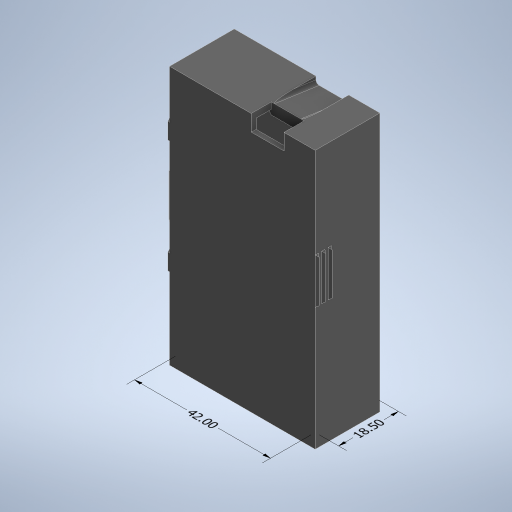
# Autodesk Inventor part: battery
Saved by Autodesk Inventor 2024.1 (Build 281209000, 209)
## iProperties
Created: 2025-03-04
Part Number: battery
Material: 一般
Document SubType Name: Modeling
Designer: hibik
Density: 1 g/cm^3
Appearance: 既定
Author: hibik
Autodesk Inventor part; units mm, degrees
sketch "スケッチ1" plane through (0, 0, 0) normal (0, 1, 0) x (-1, 0, 0)
  line L0 (-22.5, -10) -> (22.5, -10)
  line L1 (22.5, -10) -> (22.5, 10)
  line L2 (22.5, 10) -> (-22.5, 10)
  line L3 (-22.5, 10) -> (-22.5, -10)
  line L4 (-22.5, -10) -> (22.5, 10) construction
  line L5 (22.5, -10) -> (-22.5, 10) construction
  point P0 (0, 0)
  dimension "d0" = 45
  dimension "d1" = 20
  constraints: 12 end point, 2 midpoint, 2 parallel, 1 horizontal, 1 perpendicular
  measures "d0" distance of L2.end L1.end
  measures "d1" distance of L1.end L0.end
extrude "押し出し1" add sketch "スケッチ1" along normal blind 90
sketch "スケッチ2" plane through (-22.5, 0, 10) normal (0, 0, 1) x (1, 0, 0)
  line L0 (0, 0) -> (0, 90) projected
  line L1 (0, 65) -> (-3, 65)
  line L2 (-3, 65) -> (-3, 60)
  line L3 (-3, 60) -> (0, 60)
  line L4 (0, 60) -> (0, 65)
  line L5 (-3, 67.5) -> (-5, 67.5)
  line L6 (-5, 67.5) -> (-5, 57.5)
  line L7 (-5, 57.5) -> (-3, 57.5)
  line L8 (-3, 57.5) -> (-3, 67.5)
  line L9 (0, 90) -> (45, 90) projected
  point P0 (22.5, 0)
  point P1 (-5, 62.5)
  point P2 (-3, 62.5)
  point P3 (-3, 60)
  point P4 (0, 60)
  point P5 (-3, 65)
  dimension "d14" = 5
  dimension "d15" = 10
  dimension "d16" = 2
  dimension "d17" = 3
  dimension "d18" = 25
  constraints: 16 end point, 4 parallel, 2 horizontal, 2 midpoint, 2 perpendicular, 1 collinear, 1 horizontal alignment, 1 point on line
  measures "d14" distance of L1.end L2.end
  measures "d15" distance of L5.end L6.end
  measures "d16" distance of L5.start L5.end
  measures "d17" distance of L1.start L1.end
  measures "d18" distance between parallel lines of L9 L1
ref_plane "作業平面1" through (0, 45, 0) normal (0, 1, 0) x (1, 0, 0)
extrude "押し出し2" add sketch "スケッチ2" against normal up to surface (20 mm away)
mirror "ミラー1" about plane through (0, 45, 0) normal (0, 1, 0) of "押し出し2"
sketch "スケッチ3" plane through (-27.5, 67.5, 10) normal (0, 1, 0) x (1, 0, 0)
  line L0 (4.5, 0) -> (-25.5, 51.9615) projected
  line L1 (2, 20) -> (0, 20) projected
  line L2 (0, 0) -> (0, 20) projected
  line L3 (2, 0) -> (0, 0) projected
  line L4 (2, 0) -> (2, 20) projected
  line L5 (5, 20) -> (2, 20) projected
  line L6 (2, 0) -> (2, 20) projected
  line L7 (5, 0) -> (2, 0) projected
  line L8 (5, 20) -> (5, 0) projected
  point P0 (27.5, 10)
  point P1 (4.5, 0)
  point P2 (0, 7.7942)
extrude "押し出し3" cut sketch "スケッチ3" against normal through all contours L7 L4 L0 | L4 L3 L2 L0
sketch "スケッチ4" plane through (22.5, 0, 10) normal (1, 0, 0) x (0, 0, -1)
  line L0 (6.75, 92.2249) -> (6.75, 87.9989) projected
  line L1 (6.75, 87.9989) -> (1.25, 90.7989) projected
  line L2 (1.25, 92.2249) -> (1.25, 90.7989) projected
  line L3 (20, 90) -> (0, 90) projected
  line L4 (6.95, 90) -> (6.95, 87.7989)
  line L5 (6.95, 87.7989) -> (0, 87.7989)
  line L6 (0, 0) -> (0, 90) projected
  line L7 (0, 90) -> (20, 90) projected
  arc A0 (7.95, 90) -> (20, 90.2989) centre (12.7443, 139.7696) ccw
  line L8 (20, 0) -> (20, 90) projected
  point P0 (10, 0)
  point P1 (7.95, 90)
  point P2 (17.5386, 90)
  dimension "d26" = 0.2
  dimension "d27" = 0.2
  dimension "d28" = 50
  dimension "d29" = 1
  dimension "d32" = 2.5
  constraints: 4 end point, 4 point on line, 2 perpendicular, 2 point on circle, 1 centre point, 1 vertical
  measures "d26" distance from line of L0.end L5
  measures "d27" distance between parallel lines of L0 L4
  measures "d28" radius of A0
  measures "d29" distance from line of L4 A0.start
  measures "d32" distance from line of A0.end L5
extrude "押し出し4" cut sketch "スケッチ4" against normal through all
sketch "スケッチ5" plane through (22.5, 87.7989, 3.05) normal (0, 0, 1) x (1, 0, 0)
  line L0 (-36.25, 2.2011) -> (-36.25, 5.1444)
  line L1 (-30.25, 3.7011) -> (-30.25, 2.2011)
  line L2 (-24.85, 7.7011) -> (-24.85, 2.2011)
  line L3 (-20.65, 2.2011) -> (-20.65, 7.7011)
  line L4 (-24.85, 7.7011) -> (-24.85, 2.2011)
  line L5 (-15.25, 2.2011) -> (-15.25, 3.7011)
  line L6 (-9.25, 9.2011) -> (-9.25, 6.2579)
  line L7 (0, 0) -> (-45, 0)
  line L8 (-36.25, 2.2011) -> (-45, 2.2011)
  line L9 (-45, 2.2011) -> (-45, 0)
  line L10 (-45, 0) -> (-36.25, 0)
  line L11 (-36.25, 0) -> (-36.25, 2.2011)
  line L12 (-30.25, 2.2011) -> (-24.85, 2.2011)
  line L13 (-24.85, 2.2011) -> (-24.85, 0)
  line L14 (-24.85, 0) -> (-30.25, 0)
  line L15 (-30.25, 0) -> (-30.25, 2.2011)
  line L16 (-20.65, 2.2011) -> (-15.25, 2.2011)
  line L17 (-15.25, 2.2011) -> (-15.25, 0)
  line L18 (-15.25, 0) -> (-20.65, 0)
  line L19 (-20.65, 0) -> (-20.65, 2.2011)
  line L20 (-9.25, 6.2579) -> (0, 6.2579)
  line L21 (0, 6.2579) -> (0, 0)
  line L22 (0, 0) -> (-9.25, 0)
  line L23 (-9.25, 0) -> (-9.25, 6.2579)
  point P0 (-22.5, -87.7989)
  point P1 (-9.25, 0)
extrude "押し出し5" add sketch "スケッチ5" along normal up to surface (6.95 mm away)
sketch "スケッチ6" plane through (0, 0, 0) normal (0, -1, 0) x (1, 0, 0)
  line L0 (21, -8.5) -> (-21, -8.5)
  line L1 (-21, -8.5) -> (-21, 8.5)
  line L2 (-21, 8.5) -> (21, 8.5)
  line L3 (21, 8.5) -> (21, -8.5)
  line L4 (21, -8.5) -> (-21, 8.5) construction
  line L5 (-21, -8.5) -> (21, 8.5) construction
  point P0 (0, 0)
  dimension "d35" = 42
  dimension "d36" = 17
  constraints: 12 end point, 2 midpoint, 2 parallel, 1 horizontal, 1 perpendicular
  measures "d35" distance of L1.end L2.end
  measures "d36" distance of L0.end L1.end
extrude "押し出し6" cut sketch "スケッチ6" against normal blind 78
sketch "スケッチ7" plane through (-21, 0, -8.5) normal (0, 0, 1) x (1, 0, 0)
  line L0 (42, 0) -> (0, 0) projected
  line L1 (42, 0) -> (42, 78) projected
  line L2 (42, 78) -> (0, 78) projected
  line L3 (0, 0) -> (0, 78) projected
  line L4 (42, 78) -> (27, 78)
  line L5 (27, 78) -> (27, 58)
  line L6 (27, 58) -> (42, 58)
  line L7 (42, 58) -> (42, 78)
  line L8 (27, 73) -> (42, 73)
  point P0 (21, 0)
  point P1 (42, 58)
  point P2 (27, 78)
  dimension "d39" = 15
  dimension "d40" = 20
  dimension "d82" = 15
  constraints: 10 end point, 3 parallel, 3 point on line, 1 collinear, 1 horizontal, 1 perpendicular
  measures "d39" distance of L6.end L5.end
  measures "d40" distance of L5.end L4.end
  measures "d82" distance between parallel lines of L6 L8
extrude "押し出し7" cut sketch "スケッチ7" against normal through all contours L6 L5 L8 L1
sketch "スケッチ8" plane through (13.25, 94.0568, 3.05) normal (0, 1, 0) x (1, 0, 0)
  line L0 (9.25, 0) -> (9.25, -6.95) projected
  line L1 (9.25, -6.95) -> (-35.75, -6.95)
  line L2 (-35.75, -6.95) -> (-35.75, 13.05)
  line L3 (-35.75, 13.05) -> (9.25, 13.05)
  line L4 (9.25, 13.05) -> (9.25, -6.95)
  point P0 (-13.25, 3.05)
  constraints: 8 end point, 2 parallel, 1 horizontal, 1 perpendicular
ref_plane "作業平面2" through (0, 80, 0) normal (0, -1, 0) x (1, 0, 0)
extrude "押し出し8" cut sketch "スケッチ8" against normal up to surface (14.0568 mm away)
sketch "スケッチ9" plane through (-22.5, 0, 10) normal (0, 0, 1) x (1, 0, 0)
  line L0 (25.2358, 80.5) -> (25.2358, 84.3806)
  line L1 (0, 80) -> (45, 80) projected
  line L2 (25.2358, 80) -> (35.3747, 80)
  line L3 (35.3747, 80) -> (35.3747, 75)
  line L4 (35.3747, 75) -> (25.2358, 75)
  line L5 (25.2358, 75) -> (25.2358, 80)
  point P0 (22.5, 0)
  point P1 (35.3747, 80.5)
  dimension "d46" = 5
  constraints: 10 end point, 2 parallel, 2 point on line, 1 collinear, 1 horizontal, 1 perpendicular, 1 vertical, 3 other
  measures "d46" distance of L2.end L3.end
extrude "押し出し9" cut sketch "スケッチ9" against normal blind 6.2
sketch "スケッチ14" plane through (-22.5, 60, -10) normal (-1, 0, 0) x (0, 0, 1)
  line L0 (20, -30) -> (20, 0) projected
  line L1 (20, -8) -> (14, -8)
  line L2 (14, -8) -> (14, -22)
  line L3 (14, -22) -> (20, -22)
  line L4 (20, -22) -> (20, -8)
  line L5 (18, -8) -> (19, -8)
  line L6 (19, -8) -> (19, -22)
  line L7 (19, -22) -> (18, -22)
  line L8 (18, -22) -> (18, -8)
  line L9 (17, -22) -> (17, -8)
  line L10 (16, -22) -> (16, -8)
  line L11 (15, -22) -> (15, -8)
  point P0 (10, -60)
  point P1 (20, -15)
  point P2 (20, -15)
  point P3 (20, -8)
  dimension "d60" = 14
  dimension "d61" = 6
  dimension "d62" = 1
  dimension "d63" = 1
  dimension "d66" = 1
  constraints: 22 end point, 4 parallel, 3 horizontal, 2 midpoint, 2 perpendicular, 2 point on line, 1 coincident, 1 collinear, 9 other
  measures "d60" distance of L1.end L2.end
  measures "d61" distance of L1.start L1.end
  measures "d62" distance between parallel lines of L0 L6
  measures "d63" distance between parallel lines of L8 L6
  measures "d66" distance of L7.end L9.start
extrude "押し出し14" add sketch "スケッチ14" along normal blind 2 draft -35 contours L3 L6 L1 L0 | L3 L9 L1 L8 | L3 L11 L1 L10
ref_plane "作業平面3" through (0, 0, -10) normal (-1, 0, 0) x (0, 0, 1)
mirror "ミラー2" about plane through (0, 0, -10) normal (-1, 0, 0) of "押し出し14"
sketch "スケッチ16" plane through (-21, 0, -8.5) normal (0, 0, 1) x (1, 0, 0)
  line L0 (42, 0) -> (0, 0) projected
  line L1 (0, 0) -> (42, 0)
  line L2 (42, 0) -> (42, 3)
  line L3 (42, 3) -> (0, 3)
  line L4 (0, 3) -> (0, 0)
  point P0 (21, 0)
  dimension "d73" = 3
  constraints: 8 end point, 2 parallel, 1 horizontal, 1 perpendicular, 1 point on line
  measures "d73" distance of L1.end L2.end
extrude "押し出し15" cut sketch "スケッチ16" against normal through all
sketch "スケッチ17" plane through (-21, 3, -8.5) normal (0, -1, 0) x (1, 0, 0)
  line L0 (0, -1.5) -> (0, 17) projected
  line L1 (0, 17) -> (42, 17) projected
  line L2 (42, 17) -> (42, -1.5) projected
  line L3 (43.5, -1.5) -> (42, -1.5) projected
  line L4 (43.5, 18.5) -> (43.5, -1.5) projected
  line L5 (-1.5, 18.5) -> (43.5, 18.5) projected
  line L6 (-1.5, -1.5) -> (-1.5, 18.5) projected
  line L7 (0, -1.5) -> (-1.5, -1.5) projected
  line L8 (1.5, -1.5) -> (40.5, -1.5)
  line L9 (40.5, -1.5) -> (40.5, 15.5)
  line L10 (40.5, 15.5) -> (1.5, 15.5)
  line L11 (1.5, 15.5) -> (1.5, -1.5)
  line L12 (42, -1.5) -> (0, -1.5) projected
  line L13 (0, 17) -> (42, 17) projected
  point P0 (21, 8.5)
  point P1 (21, 15.5)
  point P2 (21, 17)
  point P3 (1.5, -1.5)
  point P4 (40.5, -1.5)
  dimension "d76" = 1.5
  dimension "d77" = 1.5
  constraints: 8 end point, 2 midpoint, 2 parallel, 1 collinear, 1 horizontal, 1 perpendicular, 1 vertical alignment
  measures "d76" distance between parallel lines of L1 L10
  measures "d77" distance between parallel lines of L0 L11
extrude "押し出し16" add sketch "スケッチ17" against normal blind 2 contours L0 L1 L2 L12 L9 L10 L11
sketch "スケッチ18" plane through (0, 0, 0) normal (0, -1, 0) x (1, 0, 0)
  line L0 (-19.5, -8.5) -> (19.5, -8.5) projected
  line L1 (-19.5, -8.5) -> (-19.5, 7) projected
  line L2 (-19.5, 7) -> (19.5, 7) projected
  line L3 (19.5, 7) -> (19.5, -8.5) projected
  line L4 (21, 8.5) -> (21, -10) projected
  line L5 (-21, 8.5) -> (21, 8.5) projected
  line L6 (-21, -10) -> (-21, 8.5) projected
  line L7 (21, -10) -> (-21, -10) projected
  line L8 (-19.5, -8.5) -> (-19.5, -10)
  line L9 (19.5, -8.5) -> (19.5, -10)
  point P0 (0, 0)
  constraints: 4 end point, 2 perpendicular, 2 point on line
extrude "押し出し17" add sketch "スケッチ18" against normal blind 1.6 contours L8 L7 L6 L5 L4 L9 L3 L2 L1
sketch "スケッチ19" plane through (-22.5, 0, 3.8) normal (0, 0, 1) x (1, 0, 0)
  line L0 (35.3747, 78) -> (25.2358, 78) projected
  line L1 (35.3747, 80) -> (35.3747, 78) projected
  line L2 (25.2358, 80) -> (35.3747, 80) projected
  line L3 (25.2358, 78) -> (25.2358, 80) projected
  line L4 (25.2358, 80) -> (35.3747, 80)
  line L5 (35.3747, 80) -> (35.3747, 76.5)
  line L6 (35.3747, 76.5) -> (25.2358, 76.5)
  line L7 (25.2358, 76.5) -> (25.2358, 80)
  point P0 (22.5, 0)
  dimension "d83" = 3.5
  constraints: 8 end point, 2 parallel, 1 collinear, 1 horizontal, 1 perpendicular
  measures "d83" distance of L4.end L5.end
extrude "押し出し18" add sketch "スケッチ19" against normal up to surface (12.3 mm away) contours L5 L6 L7 L0
sketch "スケッチ20" plane through (2.7358, 75, 10) normal (1, 0, 0) x (0, 0, -1)
  line L0 (6.2, 3) -> (6.2, 5) projected
  line L1 (6.2, 3) -> (6.2, 1.5) projected
  line L2 (6.2, 1.5) -> (18.5, 1.5) projected
  line L3 (18.5, 1.5) -> (18.5, 3) projected
  line L4 (18.5, -70) -> (18.5, 3) projected
  line L5 (18.5, -70) -> (18.5, -72) projected
  line L6 (18.5, -72) -> (18.5, -70) projected
  line L7 (18.5, -70) -> (18.5, -17) projected
  line L8 (18.5, -17) -> (18.5, -2) projected
  line L9 (18.5, -2) -> (18.5, 3) projected
  line L10 (18.5, 3) -> (18.5, 1.5) projected
  line L11 (6.2, 5) -> (20, 3)
  line L12 (20, -10) -> (20, 5) projected
  line L13 (6.2, 5) -> (20, 5)
  point P0 (10, -75)
  constraints: 4 end point, 1 horizontal, 1 horizontal alignment, 1 point on line
extrude "押し出し19" cut sketch "スケッチ20" along normal up to surface (10.1389 mm away)
fillet "フィレット1" radius 3 2 edges at (2.7358, 78, -2.35) (12.8747, 78, -2.35)
fillet "フィレット2" radius 1 2 edges at (2.7358, 79, -3.1) (12.8747, 79, -3.1)
sketch "スケッチ21" plane through (-21, 3, 8.5) normal (0, -1, 0) x (1, 0, 0)
  line L0 (1.5, -17) -> (40.5, -17) projected
  line L1 (1.5, -17) -> (1.5, -1.5) projected
  line L2 (1.5, -1.5) -> (40.5, -1.5) projected
  line L3 (40.5, -1.5) -> (40.5, -17) projected
  line L4 (42, 0) -> (42, -18.5) projected
  line L5 (0, 0) -> (42, 0) projected
  line L6 (0, -18.5) -> (0, 0) projected
  line L7 (42, -18.5) -> (0, -18.5) projected
  circle A0 centre (0, -16.25) radius 0.75
  circle A1 centre (42, -16.25) radius 0.75
  point P0 (21, -8.5)
  point P1 (42, -15.5)
  point P2 (42, -17)
  point P3 (0, -15.5)
  point P4 (0, -17)
  dimension "d96" = 1.5
  dimension "d97" = 1.5
  constraints: 2 centre point, 2 point on line, 2 tangent
  measures "d96" diameter of A0
  measures "d97" diameter of A1
extrude "押し出し20" cut sketch "スケッチ21" along normal up to surface (1.4 mm away) contours A1 L4 | L6 A0 picked at (42.2671, -16.4455) picked at (-0.2854, -16.4371)
equation "\"d27\" = d26"
equation "\"d63\" = d62"
equation "\"d77\" = d76"
